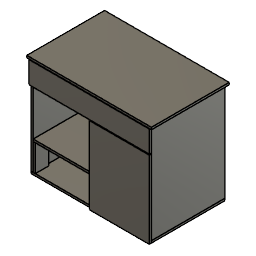
1 (Autodesk Fusion 360 design; units mm, degrees)
part number: 2026-08-15-11-16-41-561
Autodesk Fusion 360 part; units mm, degrees
other "Base Mesh Feature5"
sketch "bottom" plane through (0, 0, 0) normal (0, 1, 0) x (1, 0, 0)
  line L0 (0, 0) -> (900, 0)
  line L1 (900, 0) -> (900, -550)
  line L2 (900, -550) -> (0, -550)
  line L3 (0, -550) -> (0, 0)
  dimension "d39" = 900
  dimension "d40" = 550
  constraint horizontal L0
  constraint vertical L1
  constraint horizontal L2
  constraint vertical L3
  constraint coincident L0.start L3.end
  measures "d39" distance of L0.start L0.end
  measures "d40" distance of L0.start L2.end
extrude "Extrude6" add sketch "bottom" along normal blind 16 makes body 1
sketch "side" plane through (900, 0, 0) normal (1, 0, 0) x (0, 0, -1)
  line L0 (-550, 0) -> (0, 0)
  line L1 (0, 0) -> (0, 16)
  line L2 (0, 16) -> (-550, 16)
  line L3 (-550, 16) -> (-550, 0)
  line L4 (0, 16) -> (-550, 16)
  line L5 (-550, 16) -> (-550, 750)
  line L6 (-550, 750) -> (0, 750)
  line L7 (0, 750) -> (0, 16)
  dimension "d44" = 550
  dimension "d45" = 734
  constraint horizontal L4
  constraint vertical L5
  constraint horizontal L6
  constraint vertical L7
  constraint coincident L1.end L2.start
  measures "d44" distance of L1.end L2.end
  measures "d45" distance of L1.end L6.end
extrude "Extrude7" add sketch "side" against normal blind 16 separate body contours L2 L4 L5 L6 L7 makes body 2
sketch "side (1)" plane through (0, 0, 0) normal (-1, 0, 0) x (0, 0, 1)
  line L0 (0, 0) -> (550, 0)
  line L1 (550, 0) -> (550, 16)
  line L2 (550, 16) -> (0, 16)
  line L3 (0, 16) -> (0, 0)
  line L4 (0, 16) -> (550, 16)
  line L5 (550, 16) -> (550, 750)
  line L6 (550, 750) -> (0, 750)
  line L7 (0, 750) -> (0, 16)
  dimension "d48" = 550
  dimension "d49" = 734
  constraint horizontal L4
  constraint vertical L5
  constraint horizontal L6
  constraint vertical L7
  constraint coincident L2.end L3.start
  measures "d48" distance of L2.end L1.end
  measures "d49" distance of L2.end L6.end
extrude "Extrude8" add sketch "side (1)" against normal blind 16 separate body contours L2 L4 L5 L6 L7 makes body 3
sketch "back" plane through (0, 0, 0) normal (0, 0, -1) x (-1, 0, 0)
  line L0 (-900, 0) -> (0, 0)
  line L1 (0, 0) -> (0, 16)
  line L2 (0, 16) -> (-900, 16)
  line L3 (-900, 16) -> (-900, 0)
  line L4 (-16, 16) -> (-884, 16)
  line L5 (-884, 16) -> (-884, 750)
  line L6 (-884, 750) -> (-16, 750)
  line L7 (-16, 750) -> (-16, 16)
  point P0 (-16, 16)
  dimension "d52" = 868
  dimension "d53" = 734
  constraint horizontal L4
  constraint vertical L5
  constraint horizontal L6
  constraint vertical L7
  constraint coincident P0 L4.start
  measures "d52" distance of P0 L4.end
  measures "d53" distance of P0 L6.end
extrude "Extrude9" add sketch "back" against normal blind 16 separate body contours L2 L4 L5 L6 L7 makes body 4
sketch "doors" plane through (0, 0, 550) normal (0, 0, 1) x (1, 0, 0)
  line L0 (0, 0) -> (900, 0)
  line L1 (900, 0) -> (900, 16)
  line L2 (900, 16) -> (0, 16)
  line L3 (0, 16) -> (0, 0)
  line L4 (0, 0) -> (448, 0)
  line L5 (448, 0) -> (448, 578)
  line L6 (448, 578) -> (0, 578)
  line L7 (0, 578) -> (0, 0)
  line L8 (900, 0) -> (452, 0)
  line L9 (452, 0) -> (452, 578)
  line L10 (452, 578) -> (900, 578)
  line L11 (900, 578) -> (900, 0)
  point P0 (16, 16)
  point P1 (884, 16)
  dimension "d58" = 448
  dimension "d59" = 578
  dimension "d60" = 448
  dimension "d61" = 578
  constraint horizontal L4
  constraint vertical L5
  constraint horizontal L6
  constraint vertical L7
  constraint coincident L0.start L3.end
  constraint horizontal L8
  constraint vertical L9
  constraint horizontal L10
  constraint vertical L11
  constraint coincident L0.end L1.start
  measures "d58" distance of L0.start L4.end
  measures "d59" distance of L0.start L6.end
  measures "d60" distance of L0.end L8.end
  measures "d61" distance of L0.end L10.end
extrude "Extrude10" add sketch "doors" along normal blind 16 separate body contours L0 L2 L3 L4 L5 L7 | L2 L5 L6 L7 makes body 5
extrude "Extrude11" add sketch "doors" along normal blind 16 separate body contours L0 L1 L2 L8 L9 L11 | L2 L9 L10 L11 makes body 6
sketch "face" plane through (0, 0, 550) normal (0, 0, 1) x (1, 0, 0)
  line L0 (0, 750) -> (0, 16)
  line L1 (0, 16) -> (16, 16)
  line L2 (16, 16) -> (16, 750)
  line L3 (16, 750) -> (0, 750)
  line L4 (0, 750) -> (100, 750)
  line L5 (100, 750) -> (100, 747)
  line L6 (100, 747) -> (0, 747)
  line L7 (0, 747) -> (0, 750)
  line L8 (0, 747) -> (900, 747)
  line L9 (900, 747) -> (900, 584)
  line L10 (900, 584) -> (0, 584)
  line L11 (0, 584) -> (0, 747)
  dimension "d74" = 100
  dimension "d75" = 3
  dimension "d76" = 900
  dimension "d77" = 163
  constraint horizontal L4
  constraint vertical L5
  constraint horizontal L6
  constraint vertical L7
  constraint coincident L0.start L3.end
  constraint horizontal L8
  constraint vertical L9
  constraint horizontal L10
  constraint vertical L11
  measures "d74" distance of L0.start L4.end
  measures "d75" distance of L0.start L6.end
  measures "d76" distance of L6.end L8.end
  measures "d77" distance of L6.end L10.end
extrude "Extrude13" add sketch "face" along normal blind 16 separate body contours L0 L2 L6 L8 L10 L11 | L2 L6 L8 L9 L10 makes body 7
sketch "brace" plane through (0, 750, 0) normal (0, 1, 0) x (-1, 0, 0)
  line L0 (0, 0) -> (0, 550)
  line L1 (0, 550) -> (-16, 550)
  line L2 (-16, 550) -> (-16, 0)
  line L3 (-16, 0) -> (0, 0)
  line L4 (-16, 550) -> (-884, 550)
  line L5 (-884, 550) -> (-884, 450)
  line L6 (-884, 450) -> (-16, 450)
  line L7 (-16, 450) -> (-16, 550)
  line L8 (-16, 16) -> (-884, 16)
  line L9 (-884, 16) -> (-884, 116)
  line L10 (-884, 116) -> (-16, 116)
  line L11 (-16, 116) -> (-16, 16)
  point P0 (-16, 16)
  dimension "d80" = 868
  dimension "d81" = 100
  dimension "d82" = 868
  dimension "d83" = 100
  constraint horizontal L4
  constraint vertical L5
  constraint horizontal L6
  constraint vertical L7
  constraint coincident L1.end L2.start
  constraint horizontal L8
  constraint vertical L9
  constraint horizontal L10
  constraint vertical L11
  constraint coincident P0 L8.start
  measures "d80" distance of L1.end L4.end
  measures "d81" distance of L1.end L6.end
  measures "d82" distance of P0 L8.end
  measures "d83" distance of P0 L10.end
extrude "Extrude14" add sketch "brace" against normal blind 16 separate body contours L2 L4 L5 L6 L7 makes body 8
extrude "Extrude15" add sketch "brace" against normal blind 16 separate body contours L2 L8 L9 L10 L11 makes body 9
sketch "d_back" plane through (0, 0, 16) normal (0, 0, 1) x (1, 0, 0)
  line L0 (884, 750) -> (16, 750)
  line L1 (16, 750) -> (16, 16)
  line L2 (16, 16) -> (884, 16)
  line L3 (884, 16) -> (884, 750)
  line L4 (16, 734) -> (46, 734)
  line L5 (46, 734) -> (46, 731)
  line L6 (46, 731) -> (16, 731)
  line L7 (16, 731) -> (16, 734)
  line L8 (46, 731) -> (854, 731)
  line L9 (854, 731) -> (854, 581)
  line L10 (854, 581) -> (46, 581)
  line L11 (46, 581) -> (46, 731)
  point P0 (16, 734)
  dimension "d101" = 30
  dimension "d102" = 3
  dimension "d103" = 808
  dimension "d104" = 150
  constraint horizontal L4
  constraint vertical L5
  constraint horizontal L6
  constraint vertical L7
  constraint coincident P0 L4.start
  constraint horizontal L8
  constraint vertical L9
  constraint horizontal L10
  constraint vertical L11
  measures "d101" distance of P0 L4.end
  measures "d102" distance of P0 L6.end
  measures "d103" distance of L5.end L8.end
  measures "d104" distance of L5.end L10.end
extrude "Extrude17" add sketch "d_back" along normal blind 16 separate body contours L8 L9 L10 L11 makes body 10
sketch "d_side" plane through (854, 0, 0) normal (1, 0, 0) x (0, 0, -1)
  line L0 (-16, 581) -> (-16, 731)
  line L1 (-16, 731) -> (-32, 731)
  line L2 (-32, 731) -> (-32, 581)
  line L3 (-32, 581) -> (-16, 581)
  line L4 (-16, 731) -> (-547, 731)
  line L5 (-547, 731) -> (-547, 581)
  line L6 (-547, 581) -> (-16, 581)
  line L7 (-16, 581) -> (-16, 731)
  dimension "d107" = 531
  dimension "d108" = 150
  constraint horizontal L4
  constraint vertical L5
  constraint horizontal L6
  constraint vertical L7
  constraint coincident L0.end L1.start
  measures "d107" distance of L0.end L4.end
  measures "d108" distance of L0.end L0.start
extrude "Extrude18" add sketch "d_side" along normal blind 16 separate body makes body 11
sketch "d-side" plane through (46, 0, 0) normal (-1, 0, 0) x (0, 0, 1)
  line L0 (16, 731) -> (16, 581)
  line L1 (16, 581) -> (32, 581)
  line L2 (32, 581) -> (32, 731)
  line L3 (32, 731) -> (16, 731)
  line L4 (16, 581) -> (547, 581)
  line L5 (547, 581) -> (547, 731)
  line L6 (547, 731) -> (16, 731)
  line L7 (16, 731) -> (16, 581)
  dimension "d111" = 531
  dimension "d112" = 150
  constraint horizontal L4
  constraint vertical L5
  constraint horizontal L6
  constraint vertical L7
  constraint coincident L0.end L1.start
  measures "d111" distance of L0.end L4.end
  measures "d112" distance of L0.end L0.start
extrude "Extrude19" add sketch "d-side" along normal blind 16 separate body makes body 12
sketch "Sketch23" plane through (0, 581, 0) normal (0, -1, 0) x (1, 0, 0)
  line L0 (46, 16) -> (854, 16)
  line L1 (854, 16) -> (854, 32)
  line L2 (854, 32) -> (46, 32)
  line L3 (46, 32) -> (46, 16)
  line L4 (46, 32) -> (854, 32)
  line L5 (854, 32) -> (854, 547)
  line L6 (854, 547) -> (46, 547)
  line L7 (46, 547) -> (46, 32)
  dimension "d115" = 808
  dimension "d116" = 515
  constraint horizontal L4
  constraint vertical L5
  constraint horizontal L6
  constraint vertical L7
  constraint coincident L2.end L3.start
  measures "d115" distance of L2.end L1.end
  measures "d116" distance of L2.end L6.end
extrude "Extrude20" add sketch "Sketch23" against normal blind 16 separate body contours L2 L4 L5 L6 L7 makes body 13
sketch "top" plane through (0, 750, 0) normal (0, 1, 0) x (-1, 0, 0)
  line L0 (0, 0) -> (0, 550)
  line L1 (0, 550) -> (-16, 550)
  line L2 (-16, 550) -> (-16, 0)
  line L3 (-16, 0) -> (0, 0)
  line L4 (0, 0) -> (16, 0)
  line L5 (16, 0) -> (16, -16)
  line L6 (16, -16) -> (0, -16)
  line L7 (0, -16) -> (0, 0)
  line L8 (16, -16) -> (-916, -16)
  line L9 (-916, -16) -> (-916, 566)
  line L10 (-916, 566) -> (16, 566)
  line L11 (16, 566) -> (16, -16)
  dimension "d122" = 16
  dimension "d123" = 16
  dimension "d124" = 932
  dimension "d125" = 582
  constraint horizontal L4
  constraint vertical L5
  constraint horizontal L6
  constraint vertical L7
  constraint coincident L0.start L3.end
  constraint horizontal L8
  constraint vertical L9
  constraint horizontal L10
  constraint vertical L11
  measures "d122" distance of L0.start L4.end
  measures "d123" distance of L0.start L6.end
  measures "d124" distance of L5.end L8.end
  measures "d125" distance of L5.end L10.end
extrude "Extrude21" add sketch "top" along normal blind 16 separate body contours L0 L1 L2 L3 | L4 L7 L8 L9 L10 L11 | L4 L5 L6 L7 L8 L11 makes body 14
sketch "wedge" plane through (16, 0, 0) normal (1, 0, 0) x (0, 0, -1)
  line L0 (0, 16) -> (0, 750)
  line L1 (0, 750) -> (-550, 750)
  line L2 (-550, 750) -> (-550, 16)
  line L3 (-550, 16) -> (0, 16)
  line L4 (-550, 16) -> (-450, 16)
  line L5 (-450, 16) -> (-450, 216)
  line L6 (-450, 216) -> (-550, 216)
  line L7 (-550, 216) -> (-550, 16)
  dimension "d132" = 100
  dimension "d133" = 200
  constraint horizontal L4
  constraint vertical L5
  constraint horizontal L6
  constraint vertical L7
  constraint coincident L2.end L3.start
  measures "d132" distance of L2.end L4.end
  measures "d133" distance of L2.end L6.end
extrude "Extrude22" add sketch "wedge" along normal blind 16 separate body contours L2 L3 L4 L5 L6 L7 makes body 15
sketch "shelf" plane through (0, 216, 0) normal (0, 1, 0) x (-1, 0, 0)
  line L0 (-16, 450) -> (-16, 550)
  line L1 (-16, 550) -> (-32, 550)
  line L2 (-32, 550) -> (-32, 450)
  line L3 (-32, 450) -> (-16, 450)
  line L4 (-16, 550) -> (-884, 550)
  line L5 (-884, 550) -> (-884, 19)
  line L6 (-884, 19) -> (-16, 19)
  line L7 (-16, 19) -> (-16, 550)
  dimension "d136" = 868
  dimension "d137" = 531
  constraint horizontal L4
  constraint vertical L5
  constraint horizontal L6
  constraint vertical L7
  constraint coincident L0.end L1.start
  measures "d136" distance of L0.end L4.end
  measures "d137" distance of L0.end L6.end
extrude "Extrude23" add sketch "shelf" along normal blind 16 separate body makes body 16
hidden bodies 5
equation "width_outer = 900 mm"
equation "material_thickness = 16 mm"
equation "width_inner = width_outer - ( 2 * material_thickness )"
equation "depth_outer = 550 mm"
equation "drawer_side_gap = 14 mm"
equation "drawer_width_outer = width_inner - ( 2 * drawer_side_gap )"
equation "drawer_height_outer = 150 mm"
equation "height_outer = 750 mm"
equation "drawer_bottom_gap = 3 mm"
equation "drawer_face_height = drawer_height_outer + material_thickness - drawer_bottom_gap"
equation "door_height = height_outer - drawer_face_height - ( 3 * drawer_bottom_gap )"
equation "door_width = ( width_outer - door_gap ) / 2"
equation "door_gap = 4 mm"
equation "d39 = width_outer"
equation "d40 = depth_outer"
equation "d41 = material_thickness"
equation "height_inner = height_outer - material_thickness"
equation "d44 = depth_outer"
equation "d45 = height_inner"
equation "d46 = -material_thickness"
equation "d48 = depth_outer"
equation "d49 = height_inner"
equation "d50 = -material_thickness"
equation "d52 = width_inner"
equation "d53 = height_inner"
equation "d54 = -material_thickness"
equation "drawer_depth_outer = depth_outer - material_thickness - drawer_bottom_gap"
equation "brace_depth = 100 mm"
equation "d58 = door_width"
equation "d59 = door_height"
equation "d60 = door_width"
equation "d61 = door_height"
equation "d62 = material_thickness"
equation "d64 = material_thickness"
equation "d75 = drawer_bottom_gap"
equation "d76 = width_outer"
equation "d77 = drawer_face_height"
equation "d78 = material_thickness"
equation "d80 = width_inner"
equation "d81 = brace_depth"
equation "d82 = width_inner"
equation "d83 = brace_depth"
equation "d84 = -material_thickness"
equation "d86 = -material_thickness"
equation "drawer_width_inner = drawer_width_outer - ( 2 * material_thickness )"
equation "d101 = drawer_side_gap + material_thickness"
equation "d102 = drawer_bottom_gap"
equation "d103 = drawer_width_inner"
equation "d104 = drawer_height_outer"
equation "d105 = material_thickness"
equation "d107 = drawer_depth_outer"
equation "d108 = drawer_height_outer"
equation "d109 = material_thickness"
equation "d111 = drawer_depth_outer"
equation "d112 = drawer_height_outer"
equation "d113 = material_thickness"
equation "d115 = drawer_width_inner"
equation "d116 = drawer_depth_inner"
equation "drawer_depth_inner = drawer_depth_outer - material_thickness"
equation "d118 = -material_thickness"
equation "counter_width = width_outer + ( 2 * material_thickness )"
equation "counter_depth = depth_outer + ( 2 * material_thickness )"
equation "d122 = material_thickness"
equation "d123 = material_thickness"
equation "d124 = counter_width"
equation "d125 = counter_depth"
equation "d126 = material_thickness"
equation "stock_width = 2750 mm"
equation "stock_depth = 1830 mm"
equation "d134 = material_thickness"
equation "d136 = width_inner"
equation "d137 = drawer_depth_outer"
equation "d138 = material_thickness"
named bodies: "bottom", "side", "side (1)", "back", "door", "door (1)", "drawer_face", "brace", "brace (1)", "drawer_back", "drawer_side", "drawer_side (1)", "drawer_bottom", "top", "wedge", "shelf"
